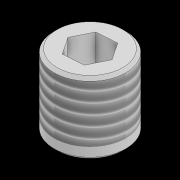
# Autodesk Inventor part: M12_HEX
Saved by Autodesk Inventor 2021 (Build 250183000, 183)
## iProperties
Created: 2024-03-28
Part Number: M12_HEX
Material: Generic
Document SubType Name: Modeling
Designer: top10
Density: 1 g/cm^3
Appearance: Default
Author: top10
Autodesk Inventor part; units mm, degrees
ref_plane "YZ Plane" through (0, 0, 0) normal (1, 0, 0) x (0, 1, 0)
ref_plane "XZ Plane" through (0, 0, 0) normal (0, 1, 0) x (-1, 0, 0)
ref_plane "XY Plane" through (0, 0, 0) normal (0, 0, 1) x (1, 0, 0)
sketch "Sketch1" plane through (0, 0, 0) normal (0, 1, 0) x (-1, 0, 0)
  circle A0 centre (0, 0) radius 6
  dimension "d3" = 12
  constraints: 1 centre point, 1 coincident
  measures "d3" diameter of A0
extrude "Extrusion1" add sketch "Sketch1" along normal mid plane 12
sketch "Sketch2" plane through (0, 6, 0) normal (0, 1, 0) x (1, 0, 0)
  line L0 (1.5326, 3.1066) -> (3.4567, 0.226)
  line L1 (3.4567, 0.226) -> (1.9241, -2.8806)
  line L2 (1.9241, -2.8806) -> (-1.5326, -3.1066)
  line L3 (-1.5326, -3.1066) -> (-3.4567, -0.226)
  line L4 (-3.4567, -0.226) -> (-1.9241, 2.8806)
  line L5 (-1.9241, 2.8806) -> (1.5326, 3.1066)
  point P0 (0, 0)
  point P1 (0, 0)
  dimension "d2" = 6
  constraints: 12 end point, 1 coincident, 13 other
  measures "d2" distance between parallel lines of L2 L5
extrude "Extrusion2" cut sketch "Sketch2" against normal blind 5.5
thread "Thread1" size "M12x1.75" class "6g" standard "ANSI Metric M Profile" length 10
chamfer "Chamfer1" distance 0.5 angle 45 2 edges at (6, 6, 0) (6, -6, 0)
body "Solid1"
